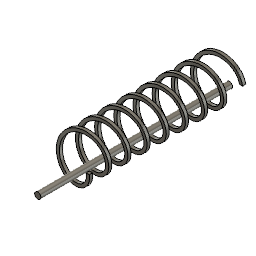
auger01 (Autodesk Fusion 360 design; units mm, degrees)
part number: 2025-12-19-00-08-44-367
Autodesk Fusion 360 part; units mm, degrees
sketch "草图1" plane through (0, 0, 0) normal (0, 0, 1) x (1, 0, 0)
  circle A0 centre (7, 7.5) radius 2.5
extrude "拉伸1" add sketch "草图1" along normal blind 150 makes body 1
coil "螺旋基本要素1" add diameter 30.698 section square size 2.5 on centre turns 8 pitch 15 right hand placed x (1, 0, 0) y (0, 1, 0) z (0, 0, 1) at (2, 13, 0) separate body makes body 2
